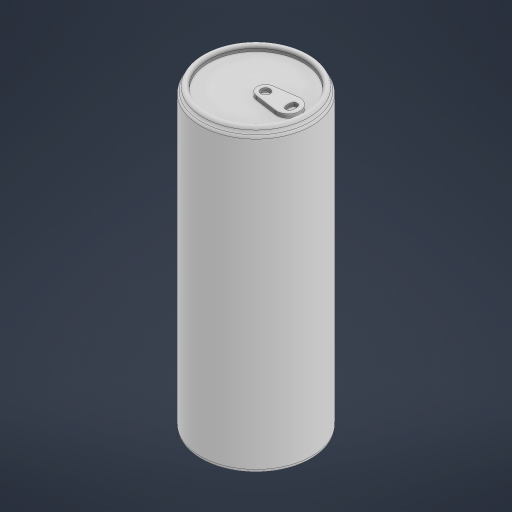
# Autodesk Inventor part: the cup
Saved by Autodesk Inventor 2024 (Build 280153000, 153)
## iProperties
Created: 2025-01-28
Part Number: the cup
Material: Generic
Document SubType Name: Modeling
Designer: turbo
Density: 1 g/cm^3
Appearance: Default
Author: turbo
Autodesk Inventor part; units mm, degrees
ref_plane "YZ Plane" through (0, 0, 0) normal (1, 0, 0) x (0, 1, 0)
ref_plane "XZ Plane" through (0, 0, 0) normal (0, 1, 0) x (-1, 0, 0)
ref_plane "XY Plane" through (0, 0, 0) normal (0, 0, 1) x (1, 0, 0)
sketch "Sketch1" plane through (0, 0, 0) normal (0, 0, 1) x (1, 0, 0)
  line L0 (30, 158) -> (30, 0) construction
  line L1 (0, 0) -> (0, 155)
  line L2 (0, 0) -> (30, 0)
  line L3 (30, 0) -> (0, 0) construction
  line L4 (0, 0) -> (0, 3) construction
  line L5 (0, 3) -> (27, 3)
  line L6 (27, 3) -> (27, 155)
  line L7 (27, 155) -> (0, 155)
  line L8 (0, 155) -> (0, 158)
  line L9 (0, 158) -> (30, 158) construction
  line L10 (27, 158) -> (27, 161) construction
  arc A0 (28.5, 159.5) -> (25.5, 159.5) centre (27, 159.5) ccw
  line L11 (28.5, 159.5) -> (28.5, 158) construction
  line L12 (25.5, 159.5) -> (25.5, 158)
  line L13 (27, 155) -> (27, 158) construction
  arc A1 (28.5, 159.5) -> (29.2857, 157.8283) centre (30.6712, 159.5) ccw
  arc A2 (30, 156.3085) -> (29.2857, 157.8283) centre (28.0261, 156.3085) ccw
  line L14 (25.5, 158) -> (0, 158)
  line L15 (30, 156.3085) -> (30, 0)
  point P0 (30, 79)
  dimension "d0" = 60
  dimension "d1" = 158
  dimension "d2" = 3
  dimension "d3" = 27
  dimension "d4" = 3
  dimension "d5" = 3
  dimension "d6" = 1.5
  constraints: 32 end point, 7 perpendicular, 7 point on circle, 5 point on line, 5 tangent, 5 vertical, 3 centre point, 3 collinear, 2 midpoint
  measures "d0" diameter of point (30, 79) L1
  measures "d1" distance of L0.start L0.end
  measures "d2" distance of L1.start L4.end
  measures "d3" distance of L4.end L5.end
  measures "d4" distance between parallel lines of L7 L9
  measures "d5" distance of L10.start L10.end
  measures "d6" radius of A0
revolve "Revolution1" add sketch "Sketch1" angle 360 about axis through (0, 0, 0) along (0, 1, 0) contours L1 L5 L6 L7 L8 L14 L12 A0 A1 A2 L15 L2
fillet "Fillet1" radius 2 1 edges at (-30, 0, 0)
sketch "Sketch2" plane through (0, 158, 0) normal (0, 1, 0) x (1, 0, 0)
  circle A0 centre (0, 0) radius 25.5 construction
  circle A1 centre (5.1723, 0) radius 4.542 construction
  circle A2 centre (17.4125, 0) radius 6.2476 construction
  line L0 (4.5394, -4.4977) -> (16.5419, -6.1866)
  line L1 (4.5394, 4.4977) -> (16.5419, 6.1866)
  arc A3 (4.5394, 4.4977) -> (4.5394, -4.4977) centre (5.1723, 0) ccw
  arc A4 (16.5419, -6.1866) -> (16.5419, 6.1866) centre (17.4125, 0) ccw
  circle A5 centre (5.1723, 0) radius 2.3915
  arc A6 (19.1723, 4.25) -> (19.1723, -4.25) centre (22.6879, 0) ccw
  arc A7 (19.1723, -4.25) -> (19.1723, 4.25) centre (15.6567, 0) ccw
  arc A8 (17.8945, -2.7286) -> (20.4501, -2.7286) centre (19.1723, 0.1434) ccw
  arc A9 (20.4501, 2.7286) -> (17.8945, 2.7286) centre (19.1723, -0.1434) ccw
  line L2 (17.8945, -2.7286) -> (17.8945, 2.7286) construction
  line L3 (20.4501, -2.7286) -> (20.4501, 2.7286) construction
  line L4 (17.4125, 0) -> (5.1723, 0) construction
  line L5 (17.1723, 0) -> (21.1723, 0) construction
  point P0 (20.4501, 0)
  point P1 (19.1723, 3)
  point P2 (19.1723, -3)
  dimension "d9" = 12.4952
  dimension "d10" = 9.084
  dimension "d11" = 17.4125
  dimension "d12" = 5.1723
  dimension "d13" = 12.2402
  dimension "d14" = 8.5
  dimension "d15" = 16
  dimension "d16" = 6
  dimension "d17" = 4
  dimension "d18" = 3.1434
  dimension "d19" = 4.783
  constraints: 24 point on circle, 12 end point, 9 centre point, 4 tangent, 3 point on line, 2 concentric, 2 equal radius, 2 horizontal, 2 parallel, 1 coincident, 1 midpoint, 1 perpendicular, 1 vertical
  measures "d9" diameter of A2
  measures "d10" diameter of A1
  measures "d11" distance of point (0, 0) A2.centre
  measures "d12" distance of point (0, 0) A1.centre
  measures "d13" distance of A2.centre A1.centre
  measures "d14" distance of A6.start A6.end
  measures "d15" distance of A1.centre L5.end
  measures "d16" distance of point (19.172, 3) point (19.172, -3)
  measures "d17" distance of L5.start L5.end
  measures "d18" radius of A8
  measures "d19" diameter of A5
extrude "Extrusion1" add sketch "Sketch2" along normal blind 2 contours A3 L1 A4 L0 | A7 A9 A6 | A8 A7 A6
body "Solid1"
